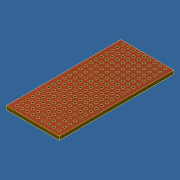
# Autodesk Inventor part: S1702_013
Saved by Autodesk Inventor 2015 SP2 (Build 190223200, 223)
## iProperties
Created: 2017-10-30
Part Number: S1702_013
Project: S1702_Circuit_Course
Material: .
Description: Plaque élec
Document SubType Name: Modeling
Designer: Benoit.CURCHOD2
Authority: brut Ø
Density: 0.001 g/cm^3
Appearance: Or
Mass: 0.00193162 g
Surface Area: 37.5236 cm^2
Volume: 1.93162 cm^3
Material number: ---
Author: Benoit.CURCHOD2
Autodesk Inventor part; units mm, degrees
ref_plane "Plan YZ" through (0, 0, 0) normal (1, 0, 0) x (0, 1, 0)
ref_plane "Plan XZ" through (0, 0, 0) normal (0, 1, 0) x (-1, 0, 0)
ref_plane "Plan XY" through (0, 0, 0) normal (0, 0, 1) x (1, 0, 0)
sketch "Esquisse9" plane through (0, 0, 0) normal (0, 0, 1) x (1, 0, 0)
  line L0 (0, 0) -> (25, 0)
  line L1 (25, 0) -> (25, 120)
  line L2 (25, 120) -> (0, 120)
  line L3 (0, 120) -> (0, 0)
  circle A0 centre (2.5, 2.5) radius 0.6
  circle A1 centre (2.5, 5) radius 0.6
  circle A2 centre (2.5, 7.5) radius 0.6
  circle A3 centre (2.5, 10) radius 0.6
  circle A4 centre (2.5, 12.5) radius 0.6
  circle A5 centre (2.5, 15) radius 0.6
  circle A6 centre (2.5, 17.5) radius 0.6
  circle A7 centre (2.5, 20) radius 0.6
  circle A8 centre (2.5, 22.5) radius 0.6
  circle A9 centre (2.5, 25) radius 0.6
  circle A10 centre (2.5, 27.5) radius 0.6
  circle A11 centre (2.5, 30) radius 0.6
  circle A12 centre (2.5, 32.5) radius 0.6
  circle A13 centre (2.5, 35) radius 0.6
  circle A14 centre (2.5, 37.5) radius 0.6
  circle A15 centre (2.5, 40) radius 0.6
  circle A16 centre (2.5, 42.5) radius 0.6
  circle A17 centre (2.5, 45) radius 0.6
  circle A18 centre (2.5, 47.5) radius 0.6
  circle A19 centre (2.5, 50) radius 0.6
  circle A20 centre (2.5, 52.5) radius 0.6
  circle A21 centre (2.5, 55) radius 0.6
  circle A22 centre (2.5, 57.5) radius 0.6
  circle A23 centre (2.5, 60) radius 0.6
  circle A24 centre (2.5, 62.5) radius 0.6
  circle A25 centre (2.5, 65) radius 0.6
  circle A26 centre (2.5, 67.5) radius 0.6
  circle A27 centre (2.5, 70) radius 0.6
  circle A28 centre (2.5, 72.5) radius 0.6
  circle A29 centre (2.5, 75) radius 0.6
  circle A30 centre (2.5, 77.5) radius 0.6
  circle A31 centre (2.5, 80) radius 0.6
  circle A32 centre (2.5, 82.5) radius 0.6
  circle A33 centre (2.5, 85) radius 0.6
  circle A34 centre (2.5, 87.5) radius 0.6
  circle A35 centre (2.5, 90) radius 0.6
  circle A36 centre (2.5, 92.5) radius 0.6
  circle A37 centre (2.5, 95) radius 0.6
  circle A38 centre (2.5, 97.5) radius 0.6
  circle A39 centre (2.5, 100) radius 0.6
  circle A40 centre (2.5, 102.5) radius 0.6
  circle A41 centre (2.5, 105) radius 0.6
  circle A42 centre (2.5, 107.5) radius 0.6
  circle A43 centre (2.5, 110) radius 0.6
  circle A44 centre (2.5, 112.5) radius 0.6
  circle A45 centre (2.5, 115) radius 0.6
  circle A46 centre (2.5, 117.5) radius 0.6
  circle A47 centre (5, 2.5) radius 0.6
  circle A48 centre (5, 5) radius 0.6
  circle A49 centre (5, 7.5) radius 0.6
  circle A50 centre (5, 10) radius 0.6
  circle A51 centre (5, 12.5) radius 0.6
  circle A52 centre (5, 15) radius 0.6
  circle A53 centre (5, 17.5) radius 0.6
  circle A54 centre (5, 20) radius 0.6
  circle A55 centre (5, 22.5) radius 0.6
  circle A56 centre (5, 25) radius 0.6
  circle A57 centre (5, 27.5) radius 0.6
  circle A58 centre (5, 30) radius 0.6
  circle A59 centre (5, 32.5) radius 0.6
  circle A60 centre (5, 35) radius 0.6
  circle A61 centre (5, 37.5) radius 0.6
  circle A62 centre (5, 40) radius 0.6
  circle A63 centre (5, 42.5) radius 0.6
  circle A64 centre (5, 45) radius 0.6
  circle A65 centre (5, 47.5) radius 0.6
  circle A66 centre (5, 50) radius 0.6
  circle A67 centre (5, 52.5) radius 0.6
  circle A68 centre (5, 55) radius 0.6
  circle A69 centre (5, 57.5) radius 0.6
  circle A70 centre (5, 60) radius 0.6
  circle A71 centre (5, 62.5) radius 0.6
  circle A72 centre (5, 65) radius 0.6
  circle A73 centre (5, 67.5) radius 0.6
  circle A74 centre (5, 70) radius 0.6
  circle A75 centre (5, 72.5) radius 0.6
  circle A76 centre (5, 75) radius 0.6
  circle A77 centre (5, 77.5) radius 0.6
  circle A78 centre (5, 80) radius 0.6
  circle A79 centre (5, 82.5) radius 0.6
  circle A80 centre (5, 85) radius 0.6
  circle A81 centre (5, 87.5) radius 0.6
  circle A82 centre (5, 90) radius 0.6
  circle A83 centre (5, 92.5) radius 0.6
  circle A84 centre (5, 95) radius 0.6
  circle A85 centre (5, 97.5) radius 0.6
  circle A86 centre (5, 100) radius 0.6
  circle A87 centre (5, 102.5) radius 0.6
  circle A88 centre (5, 105) radius 0.6
  circle A89 centre (5, 107.5) radius 0.6
  circle A90 centre (5, 110) radius 0.6
  circle A91 centre (5, 112.5) radius 0.6
  circle A92 centre (5, 115) radius 0.6
  circle A93 centre (5, 117.5) radius 0.6
  circle A94 centre (7.5, 2.5) radius 0.6
  circle A95 centre (7.5, 5) radius 0.6
  circle A96 centre (7.5, 7.5) radius 0.6
  circle A97 centre (7.5, 10) radius 0.6
  circle A98 centre (7.5, 12.5) radius 0.6
  circle A99 centre (7.5, 15) radius 0.6
  circle A100 centre (7.5, 17.5) radius 0.6
  circle A101 centre (7.5, 20) radius 0.6
  circle A102 centre (7.5, 22.5) radius 0.6
  circle A103 centre (7.5, 25) radius 0.6
  circle A104 centre (7.5, 27.5) radius 0.6
  circle A105 centre (7.5, 30) radius 0.6
  circle A106 centre (7.5, 32.5) radius 0.6
  circle A107 centre (7.5, 35) radius 0.6
  circle A108 centre (7.5, 37.5) radius 0.6
  circle A109 centre (7.5, 40) radius 0.6
  circle A110 centre (7.5, 42.5) radius 0.6
  circle A111 centre (7.5, 45) radius 0.6
  circle A112 centre (7.5, 47.5) radius 0.6
  circle A113 centre (7.5, 50) radius 0.6
  circle A114 centre (7.5, 52.5) radius 0.6
  circle A115 centre (7.5, 55) radius 0.6
  circle A116 centre (7.5, 57.5) radius 0.6
  circle A117 centre (7.5, 60) radius 0.6
  circle A118 centre (7.5, 62.5) radius 0.6
  circle A119 centre (7.5, 65) radius 0.6
  circle A120 centre (7.5, 67.5) radius 0.6
  circle A121 centre (7.5, 70) radius 0.6
  circle A122 centre (7.5, 72.5) radius 0.6
  circle A123 centre (7.5, 75) radius 0.6
  circle A124 centre (7.5, 77.5) radius 0.6
  circle A125 centre (7.5, 80) radius 0.6
  circle A126 centre (7.5, 82.5) radius 0.6
  circle A127 centre (7.5, 85) radius 0.6
  circle A128 centre (7.5, 87.5) radius 0.6
  circle A129 centre (7.5, 90) radius 0.6
  circle A130 centre (7.5, 92.5) radius 0.6
  circle A131 centre (7.5, 95) radius 0.6
  circle A132 centre (7.5, 97.5) radius 0.6
  circle A133 centre (7.5, 100) radius 0.6
  circle A134 centre (7.5, 102.5) radius 0.6
  circle A135 centre (7.5, 105) radius 0.6
  circle A136 centre (7.5, 107.5) radius 0.6
  circle A137 centre (7.5, 110) radius 0.6
  circle A138 centre (7.5, 112.5) radius 0.6
  circle A139 centre (7.5, 115) radius 0.6
  circle A140 centre (7.5, 117.5) radius 0.6
  circle A141 centre (10, 2.5) radius 0.6
  circle A142 centre (10, 5) radius 0.6
  circle A143 centre (10, 7.5) radius 0.6
  circle A144 centre (10, 10) radius 0.6
  circle A145 centre (10, 12.5) radius 0.6
  circle A146 centre (10, 15) radius 0.6
  circle A147 centre (10, 17.5) radius 0.6
  circle A148 centre (10, 20) radius 0.6
  circle A149 centre (10, 22.5) radius 0.6
  circle A150 centre (10, 25) radius 0.6
  circle A151 centre (10, 27.5) radius 0.6
  circle A152 centre (10, 30) radius 0.6
  circle A153 centre (10, 32.5) radius 0.6
  circle A154 centre (10, 35) radius 0.6
  circle A155 centre (10, 37.5) radius 0.6
  circle A156 centre (10, 40) radius 0.6
  circle A157 centre (10, 42.5) radius 0.6
  circle A158 centre (10, 45) radius 0.6
  circle A159 centre (10, 47.5) radius 0.6
  circle A160 centre (10, 50) radius 0.6
  circle A161 centre (10, 52.5) radius 0.6
  circle A162 centre (10, 55) radius 0.6
  circle A163 centre (10, 57.5) radius 0.6
  circle A164 centre (10, 60) radius 0.6
  circle A165 centre (10, 62.5) radius 0.6
  circle A166 centre (10, 65) radius 0.6
  circle A167 centre (10, 67.5) radius 0.6
  circle A168 centre (10, 70) radius 0.6
  circle A169 centre (10, 72.5) radius 0.6
  circle A170 centre (10, 75) radius 0.6
  circle A171 centre (10, 77.5) radius 0.6
  circle A172 centre (10, 80) radius 0.6
  circle A173 centre (10, 82.5) radius 0.6
  circle A174 centre (10, 85) radius 0.6
  circle A175 centre (10, 87.5) radius 0.6
  circle A176 centre (10, 90) radius 0.6
  circle A177 centre (10, 92.5) radius 0.6
  circle A178 centre (10, 95) radius 0.6
  circle A179 centre (10, 97.5) radius 0.6
  circle A180 centre (10, 100) radius 0.6
  circle A181 centre (10, 102.5) radius 0.6
  circle A182 centre (10, 105) radius 0.6
  circle A183 centre (10, 107.5) radius 0.6
  circle A184 centre (10, 110) radius 0.6
  circle A185 centre (10, 112.5) radius 0.6
  circle A186 centre (10, 115) radius 0.6
  circle A187 centre (10, 117.5) radius 0.6
  circle A188 centre (12.5, 2.5) radius 0.6
  circle A189 centre (12.5, 5) radius 0.6
  circle A190 centre (12.5, 7.5) radius 0.6
  circle A191 centre (12.5, 10) radius 0.6
  circle A192 centre (12.5, 12.5) radius 0.6
  circle A193 centre (12.5, 15) radius 0.6
  circle A194 centre (12.5, 17.5) radius 0.6
  circle A195 centre (12.5, 20) radius 0.6
  circle A196 centre (12.5, 22.5) radius 0.6
  circle A197 centre (12.5, 25) radius 0.6
  circle A198 centre (12.5, 27.5) radius 0.6
  circle A199 centre (12.5, 30) radius 0.6
  circle A200 centre (12.5, 32.5) radius 0.6
  circle A201 centre (12.5, 35) radius 0.6
  circle A202 centre (12.5, 37.5) radius 0.6
  circle A203 centre (12.5, 40) radius 0.6
  circle A204 centre (12.5, 42.5) radius 0.6
  circle A205 centre (12.5, 45) radius 0.6
  circle A206 centre (12.5, 47.5) radius 0.6
  circle A207 centre (12.5, 50) radius 0.6
  circle A208 centre (12.5, 52.5) radius 0.6
  circle A209 centre (12.5, 55) radius 0.6
  circle A210 centre (12.5, 57.5) radius 0.6
  circle A211 centre (12.5, 60) radius 0.6
  circle A212 centre (12.5, 62.5) radius 0.6
  circle A213 centre (12.5, 65) radius 0.6
  circle A214 centre (12.5, 67.5) radius 0.6
  circle A215 centre (12.5, 70) radius 0.6
  circle A216 centre (12.5, 72.5) radius 0.6
  circle A217 centre (12.5, 75) radius 0.6
  circle A218 centre (12.5, 77.5) radius 0.6
  circle A219 centre (12.5, 80) radius 0.6
  circle A220 centre (12.5, 82.5) radius 0.6
  circle A221 centre (12.5, 85) radius 0.6
  circle A222 centre (12.5, 87.5) radius 0.6
  circle A223 centre (12.5, 90) radius 0.6
  circle A224 centre (12.5, 92.5) radius 0.6
  circle A225 centre (12.5, 95) radius 0.6
  circle A226 centre (12.5, 97.5) radius 0.6
  circle A227 centre (12.5, 100) radius 0.6
  circle A228 centre (12.5, 102.5) radius 0.6
  circle A229 centre (12.5, 105) radius 0.6
  circle A230 centre (12.5, 107.5) radius 0.6
  circle A231 centre (12.5, 110) radius 0.6
  circle A232 centre (12.5, 112.5) radius 0.6
  circle A233 centre (12.5, 115) radius 0.6
  circle A234 centre (12.5, 117.5) radius 0.6
  circle A235 centre (15, 2.5) radius 0.6
  circle A236 centre (15, 5) radius 0.6
  circle A237 centre (15, 7.5) radius 0.6
  circle A238 centre (15, 10) radius 0.6
  circle A239 centre (15, 12.5) radius 0.6
  circle A240 centre (15, 15) radius 0.6
  circle A241 centre (15, 17.5) radius 0.6
  circle A242 centre (15, 20) radius 0.6
  circle A243 centre (15, 22.5) radius 0.6
  circle A244 centre (15, 25) radius 0.6
  circle A245 centre (15, 27.5) radius 0.6
  circle A246 centre (15, 30) radius 0.6
  circle A247 centre (15, 32.5) radius 0.6
  circle A248 centre (15, 35) radius 0.6
  circle A249 centre (15, 37.5) radius 0.6
  circle A250 centre (15, 40) radius 0.6
  circle A251 centre (15, 42.5) radius 0.6
  circle A252 centre (15, 45) radius 0.6
  circle A253 centre (15, 47.5) radius 0.6
  circle A254 centre (15, 50) radius 0.6
  circle A255 centre (15, 52.5) radius 0.6
  circle A256 centre (15, 55) radius 0.6
  circle A257 centre (15, 57.5) radius 0.6
  circle A258 centre (15, 60) radius 0.6
  circle A259 centre (15, 62.5) radius 0.6
  circle A260 centre (15, 65) radius 0.6
  circle A261 centre (15, 67.5) radius 0.6
  circle A262 centre (15, 70) radius 0.6
  circle A263 centre (15, 72.5) radius 0.6
  circle A264 centre (15, 75) radius 0.6
  circle A265 centre (15, 77.5) radius 0.6
  circle A266 centre (15, 80) radius 0.6
  circle A267 centre (15, 82.5) radius 0.6
  circle A268 centre (15, 85) radius 0.6
  circle A269 centre (15, 87.5) radius 0.6
  circle A270 centre (15, 90) radius 0.6
  circle A271 centre (15, 92.5) radius 0.6
  circle A272 centre (15, 95) radius 0.6
  circle A273 centre (15, 97.5) radius 0.6
  circle A274 centre (15, 100) radius 0.6
  circle A275 centre (15, 102.5) radius 0.6
  circle A276 centre (15, 105) radius 0.6
  circle A277 centre (15, 107.5) radius 0.6
  circle A278 centre (15, 110) radius 0.6
  circle A279 centre (15, 112.5) radius 0.6
  circle A280 centre (15, 115) radius 0.6
  circle A281 centre (15, 117.5) radius 0.6
  circle A282 centre (17.5, 2.5) radius 0.6
  circle A283 centre (17.5, 5) radius 0.6
  circle A284 centre (17.5, 7.5) radius 0.6
  circle A285 centre (17.5, 10) radius 0.6
  circle A286 centre (17.5, 12.5) radius 0.6
  circle A287 centre (17.5, 15) radius 0.6
  circle A288 centre (17.5, 17.5) radius 0.6
  circle A289 centre (17.5, 20) radius 0.6
  circle A290 centre (17.5, 22.5) radius 0.6
  circle A291 centre (17.5, 25) radius 0.6
  circle A292 centre (17.5, 27.5) radius 0.6
  circle A293 centre (17.5, 30) radius 0.6
  circle A294 centre (17.5, 32.5) radius 0.6
  circle A295 centre (17.5, 35) radius 0.6
  circle A296 centre (17.5, 37.5) radius 0.6
  circle A297 centre (17.5, 40) radius 0.6
  circle A298 centre (17.5, 42.5) radius 0.6
  circle A299 centre (17.5, 45) radius 0.6
  circle A300 centre (17.5, 47.5) radius 0.6
  circle A301 centre (17.5, 50) radius 0.6
  circle A302 centre (17.5, 52.5) radius 0.6
  circle A303 centre (17.5, 55) radius 0.6
  circle A304 centre (17.5, 57.5) radius 0.6
  circle A305 centre (17.5, 60) radius 0.6
  circle A306 centre (17.5, 62.5) radius 0.6
  circle A307 centre (17.5, 65) radius 0.6
  circle A308 centre (17.5, 67.5) radius 0.6
  circle A309 centre (17.5, 70) radius 0.6
  circle A310 centre (17.5, 72.5) radius 0.6
  circle A311 centre (17.5, 75) radius 0.6
  circle A312 centre (17.5, 77.5) radius 0.6
  circle A313 centre (17.5, 80) radius 0.6
  circle A314 centre (17.5, 82.5) radius 0.6
  circle A315 centre (17.5, 85) radius 0.6
  circle A316 centre (17.5, 87.5) radius 0.6
  circle A317 centre (17.5, 90) radius 0.6
  circle A318 centre (17.5, 92.5) radius 0.6
  circle A319 centre (17.5, 95) radius 0.6
  circle A320 centre (17.5, 97.5) radius 0.6
  circle A321 centre (17.5, 100) radius 0.6
  circle A322 centre (17.5, 102.5) radius 0.6
  circle A323 centre (17.5, 105) radius 0.6
  circle A324 centre (17.5, 107.5) radius 0.6
  circle A325 centre (17.5, 110) radius 0.6
  circle A326 centre (17.5, 112.5) radius 0.6
  circle A327 centre (17.5, 115) radius 0.6
  circle A328 centre (17.5, 117.5) radius 0.6
  circle A329 centre (20, 2.5) radius 0.6
  circle A330 centre (20, 5) radius 0.6
  circle A331 centre (20, 7.5) radius 0.6
  circle A332 centre (20, 10) radius 0.6
  circle A333 centre (20, 12.5) radius 0.6
  circle A334 centre (20, 15) radius 0.6
  circle A335 centre (20, 17.5) radius 0.6
  circle A336 centre (20, 20) radius 0.6
  circle A337 centre (20, 22.5) radius 0.6
  circle A338 centre (20, 25) radius 0.6
  circle A339 centre (20, 27.5) radius 0.6
  circle A340 centre (20, 30) radius 0.6
  circle A341 centre (20, 32.5) radius 0.6
  circle A342 centre (20, 35) radius 0.6
  circle A343 centre (20, 37.5) radius 0.6
  circle A344 centre (20, 40) radius 0.6
  circle A345 centre (20, 42.5) radius 0.6
  circle A346 centre (20, 45) radius 0.6
  circle A347 centre (20, 47.5) radius 0.6
  circle A348 centre (20, 50) radius 0.6
  circle A349 centre (20, 52.5) radius 0.6
  circle A350 centre (20, 55) radius 0.6
  circle A351 centre (20, 57.5) radius 0.6
  circle A352 centre (20, 60) radius 0.6
  circle A353 centre (20, 62.5) radius 0.6
  circle A354 centre (20, 65) radius 0.6
  circle A355 centre (20, 67.5) radius 0.6
  circle A356 centre (20, 70) radius 0.6
  circle A357 centre (20, 72.5) radius 0.6
  circle A358 centre (20, 75) radius 0.6
  circle A359 centre (20, 77.5) radius 0.6
  circle A360 centre (20, 80) radius 0.6
  circle A361 centre (20, 82.5) radius 0.6
  circle A362 centre (20, 85) radius 0.6
  circle A363 centre (20, 87.5) radius 0.6
  circle A364 centre (20, 90) radius 0.6
  circle A365 centre (20, 92.5) radius 0.6
  circle A366 centre (20, 95) radius 0.6
  circle A367 centre (20, 97.5) radius 0.6
  circle A368 centre (20, 100) radius 0.6
  circle A369 centre (20, 102.5) radius 0.6
  circle A370 centre (20, 105) radius 0.6
  circle A371 centre (20, 107.5) radius 0.6
  circle A372 centre (20, 110) radius 0.6
  circle A373 centre (20, 112.5) radius 0.6
  circle A374 centre (20, 115) radius 0.6
  circle A375 centre (20, 117.5) radius 0.6
  circle A376 centre (22.5, 2.5) radius 0.6
  circle A377 centre (22.5, 5) radius 0.6
  circle A378 centre (22.5, 7.5) radius 0.6
  circle A379 centre (22.5, 10) radius 0.6
  circle A380 centre (22.5, 12.5) radius 0.6
  circle A381 centre (22.5, 15) radius 0.6
  circle A382 centre (22.5, 17.5) radius 0.6
  circle A383 centre (22.5, 20) radius 0.6
  circle A384 centre (22.5, 22.5) radius 0.6
  circle A385 centre (22.5, 25) radius 0.6
  circle A386 centre (22.5, 27.5) radius 0.6
  circle A387 centre (22.5, 30) radius 0.6
  circle A388 centre (22.5, 32.5) radius 0.6
  circle A389 centre (22.5, 35) radius 0.6
  circle A390 centre (22.5, 37.5) radius 0.6
  circle A391 centre (22.5, 40) radius 0.6
  circle A392 centre (22.5, 42.5) radius 0.6
  circle A393 centre (22.5, 45) radius 0.6
  circle A394 centre (22.5, 47.5) radius 0.6
  circle A395 centre (22.5, 50) radius 0.6
  circle A396 centre (22.5, 52.5) radius 0.6
  circle A397 centre (22.5, 55) radius 0.6
  circle A398 centre (22.5, 57.5) radius 0.6
  circle A399 centre (22.5, 60) radius 0.6
  circle A400 centre (22.5, 62.5) radius 0.6
  circle A401 centre (22.5, 65) radius 0.6
  circle A402 centre (22.5, 67.5) radius 0.6
  circle A403 centre (22.5, 70) radius 0.6
  circle A404 centre (22.5, 72.5) radius 0.6
  circle A405 centre (22.5, 75) radius 0.6
  circle A406 centre (22.5, 77.5) radius 0.6
  circle A407 centre (22.5, 80) radius 0.6
  circle A408 centre (22.5, 82.5) radius 0.6
  circle A409 centre (22.5, 85) radius 0.6
  circle A410 centre (22.5, 87.5) radius 0.6
  circle A411 centre (22.5, 90) radius 0.6
  circle A412 centre (22.5, 92.5) radius 0.6
  circle A413 centre (22.5, 95) radius 0.6
  circle A414 centre (22.5, 97.5) radius 0.6
  circle A415 centre (22.5, 100) radius 0.6
  circle A416 centre (22.5, 102.5) radius 0.6
  circle A417 centre (22.5, 105) radius 0.6
  circle A418 centre (22.5, 107.5) radius 0.6
  circle A419 centre (22.5, 110) radius 0.6
  circle A420 centre (22.5, 112.5) radius 0.6
  circle A421 centre (22.5, 115) radius 0.6
  circle A422 centre (22.5, 117.5) radius 0.6
  dimension "d40" = 120
  dimension "d41" = 25
  dimension "d42" = 1.2
  dimension "d43" = 2.5
  dimension "d44" = 2.5
  dimension "d47" = 2.5
  dimension "d50" = 2.5
  constraints: 423 centre point, 8 end point, 2 horizontal, 2 parallel, 1 perpendicular, 1 vertical, 844 other
  measures "d40" distance of L0.end L1.end
  measures "d41" distance of L1.end L2.end
  measures "d42" diameter of A0
  measures "d43" distance from line of L0 A0.centre
  measures "d44" distance from line of L3 A0.centre
  measures "d47" distance of A0.centre A1.centre
  measures "d50" distance of A0.centre A47.centre
extrude "Extrusion4" add sketch "Esquisse9" along normal blind 1.7
sketch "Esquisse10" plane through (0, 0, 1.7) normal (0, 0, 1) x (1, 0, 0)
  line L0 (25, 0) -> (25, 120) projected
  line L1 (0, 120) -> (25, 120)
  line L2 (25, 120) -> (25, 54)
  line L3 (25, 54) -> (0, 54)
  line L4 (0, 54) -> (0, 120)
  line L5 (0, 0) -> (25, 0) projected
  dimension "d55" = 54
  constraints: 8 end point, 2 parallel, 1 horizontal, 1 perpendicular, 1 point on line
  measures "d55" distance between parallel lines of L5 L3
extrude "Extrusion5" cut sketch "Esquisse10" against normal through all
